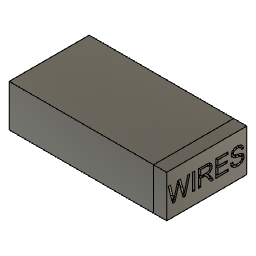
_Tattu 3S 450mah battery.8d6e4e41-cfbc-432f-a20e-b71eb7b33fd3 (Autodesk Fusion 360 design; units mm, degrees)
Autodesk Fusion 360 part; units mm, degrees
sketch "Sketch1" plane through (0, 0, 0) normal (0, 0, 1) x (1, 0, 0)
  line L0 (-27.5, 15.25) -> (27.5, 15.25)
  line L1 (27.5, 15.25) -> (27.5, -15.25)
  line L2 (27.5, -15.25) -> (-27.5, -15.25)
  line L3 (-27.5, -15.25) -> (-27.5, 15.25)
  line L4 (-27.5, 15.25) -> (27.5, -15.25) construction
  line L5 (27.5, 15.25) -> (-27.5, -15.25) construction
  line L6 (27.5, 15.25) -> (32.5, 15.25)
  line L7 (32.5, 15.25) -> (32.5, -15.25)
  line L8 (32.5, -15.25) -> (27.5, -15.25)
  dimension "d1" = 30.5
  dimension "d2" = 55
  dimension "d5" = 5
  constraint horizontal L0
  constraint vertical L1
  constraint horizontal L2
  constraint vertical L3
  constraint coincident origin L4
  constraint coincident origin L5
  constraint perpendicular L1 L6
  constraint perpendicular L0 L7
  constraint perpendicular L1 L8
  measures "d1" distance of L0.end L1.end
  measures "d2" distance of L0.start L0.end
  measures "d5" distance of L0.end L6.end
extrude "Extrude1" add sketch "Sketch1" along normal mid plane 16 contours L0 L1 L2 L3 makes body 1
extrude "Extrude2" add sketch "Sketch1" along normal mid plane 16 separate body contours L1 L6 L7 L8 makes body 2
sketch "Sketch2" plane through (32.5, 0, 0) normal (1, 0, 0) x (0, 1, 0)
  line L0 (15.25, -8) -> (15.25, 8)
  line L1 (15.25, 8) -> (-15.25, 8)
  line L2 (-15.25, 8) -> (-15.25, -8)
  line L3 (-15.25, -8) -> (15.25, -8)
  line L4 (-14.7067, -3.4864) -> (14.2138, -3.4864) construction
  line L5 (14.2138, -3.4864) -> (14.2138, 5.5136) construction
  line L6 (14.2138, 5.5136) -> (-14.7067, 5.5136) construction
  line L7 (-14.7067, 5.5136) -> (-14.7067, -3.4864) construction
  text T0 "WIRES" font "Arial" height 9 align ink ink in box 0 x 0 at (-14.6967, -3.4664) x (1, 0) y (0, 1) spacing 1 height is em
  constraint perpendicular L4 L5
  constraint parallel L4 L6
  constraint parallel L5 L7
extrude "Extrude3" cut sketch "Sketch2" against normal blind 1 text T0 bodies 2
